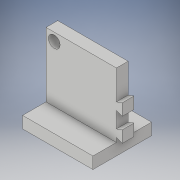
# Autodesk Inventor part: SpoolWinderDriveBase
Saved by Autodesk Inventor 2019 (Build 230136000, 136)
## iProperties
Created: 2019-01-14
Part Number: SpoolWinderDriveBase
Material: Generic
Document SubType Name: Modeling
Designer: Kepler
Density: 1 g/cm^3
Appearance: Default
Author: Kepler
Autodesk Inventor part; units mm, degrees
ref_plane "YZ Plane" through (0, 0, 0) normal (1, 0, 0) x (0, 1, 0)
ref_plane "XZ Plane" through (0, 0, 0) normal (0, 1, 0) x (-1, 0, 0)
ref_plane "XY Plane" through (0, 0, 0) normal (0, 0, 1) x (1, 0, 0)
sketch "Sketch1" plane through (0, 0, 0) normal (0, 0, 1) x (1, 0, 0)
  line L0 (0, 0) -> (0, 65)
  line L1 (0, 65) -> (60, 65)
  line L2 (60, 0) -> (0, 0)
  line L3 (60, 13.6397) -> (65, 11.8199)
  line L4 (65, 11.8199) -> (65, 21.8199)
  line L5 (65, 21.8199) -> (60, 20)
  line L6 (60, 13.6397) -> (60, 0)
  line L7 (60, 40) -> (65, 41.8199)
  line L8 (65, 41.8199) -> (65, 31.8199)
  line L9 (65, 31.8199) -> (60, 33.6397)
  line L10 (60, 65) -> (60, 40)
  line L11 (60, 33.6397) -> (60, 20)
  circle A0 centre (7, 58) radius 5
  dimension "d0" = 65
  dimension "d1" = 60
  dimension "d2" = 10
  dimension "d6" = 6.3603
  dimension "d7" = 5
  dimension "d8" = 20
  dimension "d10" = 70
  dimension "d11" = 13.6397
  dimension "d12" = 10
  dimension "d13" = 70
  dimension "d14" = 70
  dimension "d15" = 70
  dimension "d16" = 5
  dimension "d17" = 40
  dimension "d18" = 10
  dimension "d19" = 7
  dimension "d20" = 7
  constraints: 24 end point, 8 perpendicular, 2 collinear, 2 vertical, 1 centre point
  measures "d0" distance of L0.start L0.end
  measures "d1" distance of L0.end L1.end
  measures "d2" distance of L3.end L4.end
  measures "d6" distance of L3.start L5.end
  measures "d7" distance from line of L6 L3.end
  measures "d8" distance of L2.start L5.end
  measures "d10" angle of L6 L3
  measures "d11" distance of L2.start L3.start
  measures "d12" distance of L7.end L8.end
  measures "d13" angle of L10 L7
  measures "d14" angle of L11 L9
  measures "d15" angle of L5 L11
  measures "d16" distance from line of L11 L8.end
  measures "d17" distance of L2.start L7.start
  measures "d18" diameter of A0
  measures "d19" distance from line of L1 A0.centre
  measures "d20" distance from line of L0 A0.centre
extrude "Extrusion1" add sketch "Sketch1" along normal blind 10
sketch "Sketch2" plane through (0, 0, 0) normal (0, 0, -1) x (-1, 0, 0)
  line L0 (0, 65) -> (0, 0) projected
  line L1 (0, 0) -> (0, 10)
  line L2 (0, 10) -> (-60, 10)
  line L3 (-60, 0) -> (-60, 13.6397) projected
  line L4 (-60, 0) -> (0, 0)
  dimension "d23" = 10
  constraints: 6 end point, 2 point on line, 1 parallel, 1 perpendicular
  measures "d23" distance of L0.end L1.end
sketch "Sketch3" plane through (0, 0, 0) normal (0, 0, -1) x (-1, 0, 0)
  point P0 (0, 0)
extrude "Extrusion2" add sketch "Sketch2" along normal blind 20
fillet "Fillet1" radius 3 1 edges at (30, 10, 0)
sketch "Sketch4" plane through (0, 0, 10) normal (0, 0, 1) x (1, 0, 0)
  line L0 (0, 0) -> (0, 10) projected
  line L1 (60, 10) -> (60, 13) projected
  line L2 (0, 10) -> (60, 10)
  line L3 (60, 10) -> (60, 0)
  line L4 (0, 0) -> (60, 0) projected
  line L5 (60, 0) -> (0, 0)
  line L6 (0, 0) -> (0, 10)
  constraints: 8 end point, 2 perpendicular, 1 collinear, 1 horizontal
extrude "Extrusion3" add sketch "Sketch4" along normal blind 20
body "Solid1"
